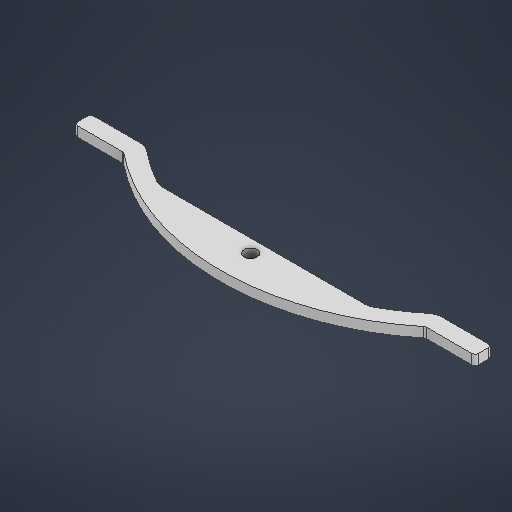
# Autodesk Inventor part: Pieza Contramolde
Saved by Autodesk Inventor 2026.2 (Build 302298000, 298)
## iProperties
Created: 2026-02-26
Part Number: Pieza Contramolde
Material: Generic
Document SubType Name: Modeling
Designer: 06aar
Density: 1 g/cm^3
Appearance: Default
Author: 06aar
Autodesk Inventor part; units mm, degrees
ref_plane "YZ Plane" through (0, 0, 0) normal (1, 0, 0) x (0, 1, 0)
ref_plane "XZ Plane" through (0, 0, 0) normal (0, 1, 0) x (-1, 0, 0)
ref_plane "XY Plane" through (0, 0, 0) normal (0, 0, 1) x (1, 0, 0)
sketch "Sketch1" plane through (0, 0, 0) normal (0, 1, 0) x (-1, 0, 0)
  circle A0 centre (0, 0) radius 75
  line L0 (0, 0) -> (45.6571, 59.5015)
  line L1 (0, 0) -> (-45.6571, 59.5015)
  line L2 (0, 0) -> (0, 75)
  circle A1 centre (0, 0) radius 72.3
  circle A2 centre (0, 0) radius 91
  line L3 (45.6571, 59.5015) -> (45.6571, 56.06)
  line L4 (45.6571, 56.06) -> (60.6571, 56.06)
  line L5 (45.6571, 59.5015) -> (45.6571, 78.7174)
  line L6 (60.6571, 56.06) -> (60.6571, 61.06)
  line L7 (60.6571, 61.06) -> (45.6571, 61.06)
  line L8 (-45.6571, 59.5015) -> (-45.6571, 56.06)
  line L9 (-45.6571, 56.06) -> (-60.6571, 56.06)
  line L10 (-45.6571, 59.5015) -> (-45.6571, 78.7174)
  line L11 (-60.6571, 56.06) -> (-60.6571, 61.06)
  line L12 (-60.6571, 61.06) -> (-45.6571, 61.06)
  line L13 (45.6571, 56.06) -> (60.6571, 56.06)
  line L14 (60.6571, 56.06) -> (60.6571, 51.06)
  line L15 (60.6571, 51.06) -> (45.6571, 51.06)
  line L16 (45.6571, 51.06) -> (45.6571, 56.06)
  circle A3 centre (0, 0) radius 67.3
  line L17 (45.6571, 51.06) -> (43.8426, 51.06)
  line L18 (-45.6571, 56.06) -> (-60.6571, 56.06)
  line L19 (-60.6571, 56.06) -> (-60.6571, 51.06)
  line L20 (-60.6571, 51.06) -> (-45.6571, 51.06)
  line L21 (-45.6571, 51.06) -> (-45.6571, 56.06)
  line L22 (-45.6571, 51.06) -> (-43.8426, 51.06)
  point P0 (44.0135, 57.3594)
  point P1 (-44.0135, 57.3594)
  dimension "d0" = 150
  dimension "d1" = 37.5
  dimension "d2" = 37.5
  dimension "d3" = 2.7
  dimension "d9" = 16
  dimension "d21" = 15
  dimension "d22" = 5
  dimension "d37" = 5
  dimension "d38" = 5
  constraints: 46 end point, 9 symmetric about line, 8 point on circle, 5 vertical, 4 coincident, 4 point on line, 3 centre point, 3 horizontal, 2 parallel, 2 perpendicular, 1 collinear, 1 concentric, 3 other
  measures "d0" diameter of A0
  measures "d1" angle of L1 L2
  measures "d2" angle of L2 L0
  measures "d3" radial gap between concentric circles of A0 A1
  measures "d9" radial gap between concentric circles of A2 A0
  measures "d21" distance of L3.end L4.end
  measures "d22" distance between parallel lines of L4 L7
  measures "d37" distance between parallel lines of L4 L15
extrude "Extrusion1" add sketch "Sketch1" along normal blind 3 contours L4 L14 L15 A0 | A0 L15 A1 L4 | A1 L16 L17 A3 L0 | L0 A3 L2 A1 | A1 L15 L16 | L2 A3 L1 A1 | L9 A1 L20 A0 | A0 L20 L19 L9 | L1 A3 L22 L21 A1 | L21 L20 A1
fillet "Fillet10" radius 1 6 edges at (-60.6571, 1.5, 56.06) (-60.6571, 1.5, 51.06) (-45.6571, 1.5, 56.06) (45.6571, 1.5, 56.06) (60.6571, 1.5, 56.06) (60.6571, 1.5, 51.06)
fillet "Fillet11" radius 5 2 edges at (-43.8426, 1.5, 51.06) (43.8426, 1.5, 51.06)
sketch "Sketch4" plane through (0, 3, 0) normal (0, 1, 0) x (1, 0, 0)
  arc A0 (-42.4996, -52.1831) -> (42.4996, -52.1831) centre (0, 0) ccw projected
  line L0 (0, -67.3) -> (0, -59.3)
  line L1 (0, -59.3) -> (31.8245, -59.3)
  line L2 (0, -59.3) -> (-31.8245, -59.3)
  circle A1 centre (0, -63.3) radius 2
  dimension "d41" = 8
  dimension "d44" = 4
  dimension "d45" = 4
  constraints: 6 end point, 2 point on circle, 1 centre point, 1 horizontal, 1 midpoint, 1 perpendicular, 1 symmetric about line, 1 vertical
  measures "d41" distance of L0.start L0.end
  measures "d44" diameter of A1
  measures "d45" distance from line of L1 A1.centre
extrude "Extrusion4" add sketch "Sketch4" against normal blind 3 contours L2 L0 A1 A0 | L0 A1 L1 A0
fillet "Fillet12" radius 5 2 edges at (-31.8245, 1.5, 59.3) (31.8245, 1.5, 59.3)
body "Solid1"
